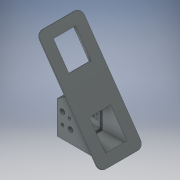
# Autodesk Inventor part: FingerScanTest
Saved by Autodesk Inventor 2017 (Build 210142000, 142)
## iProperties
Part Number: FingerScanTest
Material: Пластик АБС
Document SubType Name: Modeling
Designer: yulia_000
Density: 1.06 g/cm^3
Appearance: Цинк
Mass: 25.2515 g
Surface Area: 166.652 cm^2
Volume: 23.8222 cm^3
Author: yulia_000
Autodesk Inventor part; units mm, degrees
ref_plane "YZ Plane" through (0, 0, 0) normal (1, 0, 0) x (0, 1, 0)
sketch "Эскиз1" plane through (0, 0, 0) normal (0, 0, 1) x (1, 0, 0)
  line L0 (0, 25.2) -> (20.185268, 25.2)
  line L1 (20.185268, 25.2) -> (20.185268, 23.5) construction
  line L2 (20.185268, 23.5) -> (22.685268, 23.5) construction
  line L3 (22.685268, 23.5) -> (22.685268, 25.2) construction
  line L4 (31.435268, 25.2) -> (47.4, 2.4)
  line L5 (47.4, 2.4) -> (47.4, 0)
  line L6 (47.4, 0) -> (0, 0)
  line L7 (22.685268, 25.2) -> (31.435268, 25.2)
  line L8 (0, 25.2) -> (0, 0)
  line L9 (20.185268, 25.2) -> (22.685268, 25.2)
  point P0 (21.435268, 23.5)
  dimension "d2" = 2.4
  dimension "d8" = 1.7
  dimension "d10" = 47.4
  dimension "d13" = 25.2
  dimension "d34" = 35
  dimension "d37" = 2.5
  dimension "d38" = 10
  constraints: 21 end point, 6 perpendicular, 1 collinear, 1 horizontal, 1 midpoint, 1 parallel, 1 point on line, 1 vertical alignment
  measures "d2" distance of L4.end L5.end
  measures "d8" distance of L0.end L1.end
  measures "d10" distance of L5.end L6.end
  measures "d13" distance between parallel lines of L6 L0
  measures "d34" angle of L4 L5
  measures "d37" distance between parallel lines of L3 L1
  measures "d38" horizontal distance of L4.start point (21.435, 23.5)
extrude "Выдавливание1" add sketch "Эскиз1" along normal mid plane 21
shell "Оболочка1" thickness 3.8 outward yes removed faces 1 at (42.078423, 10, 3.5)
sketch "Эскиз7" plane through (-3.8, 29, 14.3) normal (0, 1, 0) x (1, 0, 0)
  line L0 (32.574479, 0) -> (0, 0)
  line L1 (0, 28.6) -> (32.574479, 28.6)
  line L2 (24.535268, 2) -> (27.435268, 2)
  line L3 (27.435268, 2) -> (27.435268, 26.6)
  line L4 (27.435268, 26.6) -> (24.535268, 26.6)
  line L5 (24.535268, 26.6) -> (24.535268, 2)
  line L6 (35.235268, 3.8) -> (35.235268, 24.8)
  point P0 (3.8, 14.3)
  dimension "d40" = 7.8
  dimension "d41" = 2
  dimension "d42" = 2
  dimension "d43" = 2.9
  constraints: 8 end point, 2 parallel, 1 horizontal, 1 perpendicular
  measures "d40" distance between parallel lines of L6 L3
  measures "d41" distance between parallel lines of L1 L4
  measures "d42" distance between parallel lines of L0 L2
  measures "d43" distance between parallel lines of L3 L5
extrude "Выдавливание7" cut sketch "Эскиз7" against normal blind 29
sketch "Эскиз8" plane through (0, 0, 14.3) normal (0, 0, 1) x (1, 0, 0)
  line L0 (51.2, -3.8) -> (51.2, -3.026962)
  line L1 (51.2, -3.8) -> (51.741287, -3.8)
  line L2 (51.2, -3.026962) -> (51.741287, -3.8)
  point P0 (0, 0)
  dimension "d46" = 35
  constraints: 4 end point, 1 horizontal
  measures "d46" angle of L0 L2
extrude "Выдавливание8" add sketch "Эскиз8" against normal blind 28.6
sketch "Эскиз10" plane through (0, 0, 14.3) normal (0, 0, 1) x (1, 0, 0)
  line L0 (-3.8, -3.8) -> (51.741287, -3.8)
  line L1 (52.667314, -6.691607) -> (50.64259, -3.8)
  line L2 (28.774479, 29) -> (-3.8, 29)
  line L3 (-10.124775, 84.553893) -> (-10.943927, 83.980316)
  line L4 (-10.943927, 83.980316) -> (27.553705, 29)
  line L5 (53.404551, -6.175388) -> (52.667314, -6.691607)
  line L6 (51.741287, -3.8) -> (28.774479, 29)
  line L7 (50.64259, -3.8) -> (51.741287, -3.8)
  line L8 (27.553705, 29) -> (28.774479, 29)
  line L9 (-3.8, 29) -> (28.774479, 29)
  line L10 (-10.124775, 84.553893) -> (28.774479, 29)
  line L11 (51.741287, -3.8) -> (53.404551, -6.175388)
  point P0 (0, 0)
  point P1 (23.635268, 29)
  dimension "d62" = 1
  dimension "d123" = 3.53
  dimension "d124" = 0.9
  dimension "d126" = 110.76
  constraints: 16 end point, 4 parallel, 2 collinear, 2 point on line, 1 perpendicular
  measures "d62" distance of L3.start L3.end
  measures "d123" distance of L1.start L1.end
  measures "d124" distance between parallel lines of L1 L6
  measures "d126" distance between parallel lines of L3 L5
extrude "Выдавливание9" add sketch "Эскиз10" against normal blind 28.6 contours L0 L11 L5 L1
extrude "Выдавливание10" add sketch "Эскиз10" against normal blind 28.6 contours L2 L4 L3 L10
sketch "Эскиз14" plane through (0, 0, 14.3) normal (0, 0, 1) x (1, 0, 0)
  line L0 (53.404551, -6.175388) -> (-10.124775, 84.553893)
  line L1 (-10.124775, 84.553893) -> (-10.943927, 83.980316)
  line L2 (27.553705, 29) -> (-10.943927, 83.980316)
  line L3 (53.404551, -6.175388) -> (52.667314, -6.691607)
  line L4 (-10.943927, 83.980316) -> (52.585399, -6.748964)
  line L5 (52.667314, -6.691607) -> (53.404551, -6.175388)
  line L6 (53.404551, -6.175388) -> (-10.124775, 84.553893)
  line L7 (-10.124775, 84.553893) -> (-10.943927, 83.980316)
  point P0 (0, 0)
  constraints: 8 end point, 1 collinear, 1 perpendicular
sketch "Эскиз14 outline for Выдавливание13" plane through (0, 0, 14.3) normal (0, 0, 1) x (1, 0, 0)
  line L0 (-10.943927, 83.980316) -> (52.667314, -6.691607)
  line L1 (-10.124775, 84.553893) -> (-10.943927, 83.980316)
  line L2 (53.404551, -6.175388) -> (-10.124775, 84.553893)
  line L3 (52.667314, -6.691607) -> (53.404551, -6.175388)
extrude "Выдавливание13" add sketch "Эскиз14 outline for Выдавливание13" along normal blind 8
sketch "Эскиз15" plane through (0, 0, -14.3) normal (0, 0, -1) x (-1, 0, 0)
  line L0 (10.943927, 83.980316) -> (10.124775, 84.553893)
  line L1 (10.124775, 84.553893) -> (-53.404551, -6.175388)
  line L2 (-53.404551, -6.175388) -> (-52.667314, -6.691607)
  line L3 (10.943927, 83.980316) -> (-52.667314, -6.691607)
  line L4 (-52.667314, -6.691607) -> (-53.404551, -6.175388)
  line L5 (-53.404551, -6.175388) -> (10.124775, 84.553893)
  line L6 (10.943927, 83.980316) -> (10.124775, 84.553893)
  point P0 (0, 0)
  constraints: 8 end point, 2 collinear, 1 perpendicular
extrude "Выдавливание14" add sketch "Эскиз15" along normal blind 8
fillet "Сопряжение2" radius 6 2 edges at (53.0359, -6.4335, 22.3) (53.0359, -6.4335, -22.3)
sketch "Эскиз16" plane through (0, 0, -10.5) normal (1, 0, 0) x (0, 0, -1)
  line L0 (-21, 0) -> (0, 0) projected
  line L1 (0, 0) -> (0, 25.2) projected
  line L2 (0, 25.2) -> (-21, 25.2) projected
  line L3 (-21, 25.2) -> (-21, 0) projected
  point P0 (-10.5, 0)
extrude "Выдавливание15" cut sketch "Эскиз16" against normal through all
sketch "Эскиз19" plane through (-3.8, -3.8, 14.3) normal (-1, 0, 0) x (0, 0, 1)
  line L0 (-24.8, 3.8) -> (-24.8, 29) projected
  line L1 (-24.8, 29) -> (-3.8, 29) projected
  line L2 (-3.8, 29) -> (-3.8, 3.8) projected
  line L3 (-3.8, 3.8) -> (-24.8, 3.8) projected
  line L4 (-3.55, 29.25) -> (-25.05, 29.25)
  line L5 (-25.05, 29.25) -> (-25.05, 3.55)
  line L6 (-25.05, 3.55) -> (-3.55, 3.55)
  line L7 (-3.55, 3.55) -> (-3.55, 29.25)
  point P0 (-14.3, 3.8)
  dimension "d106" = 0.25
  constraints: 8 end point, 3 other
  measures "d106" distance between parallel lines of L1 L4
extrude "Выдавливание17" cut sketch "Эскиз19" against normal up to surface (51.2 mm away)
sketch "Эскиз20" plane through (20.735268, 0, -12.3) normal (0, 1, 0) x (1, 0, 0)
  line L0 (0, -1.55) -> (2.9, -1.55) projected
  line L1 (2.9, 0) -> (2.9, -1.55) projected
  line L2 (0, 0) -> (2.9, 0) projected
  line L3 (0, -1.55) -> (0, 0) projected
  line L4 (2.9, -23.05) -> (0, -23.05) projected
  line L5 (0, -24.6) -> (0, -23.05) projected
  line L6 (2.9, -24.6) -> (0, -24.6) projected
  line L7 (2.9, -23.05) -> (2.9, -24.6) projected
  point P0 (-20.735268, -12.3)
extrude "Выдавливание18" cut sketch "Эскиз20" against normal up to surface (0.25 mm away)
sketch "Эскиз21" plane through (47.4, -0.25, -10.75) normal (-1, 0, 0) x (0, 0, 1)
  line L0 (0, 2.65) -> (21.5, 2.65) projected
  line L1 (0, 2.65) -> (0, 0) projected
  line L2 (0, 0) -> (21.5, 0) projected
  line L3 (21.5, 0) -> (21.5, 2.65) projected
  point P0 (10.75, 0.25)
extrude "Выдавливание19" cut sketch "Эскиз21" against normal blind 0.2
sketch "Эскиз22" plane through (-3.8, -3.8, 14.3) normal (-1, 0, 0) x (0, 0, 1)
  line L0 (-3.55, 29.25) -> (-3.55, 3.55) projected
  line L1 (-3.55, 3.55) -> (-25.05, 3.55) projected
  line L2 (-25.05, 3.55) -> (-25.05, 29.25) projected
  line L3 (-25.05, 29.25) -> (-3.55, 29.25) projected
  line L4 (0, 0) -> (-28.6, 0) projected
  line L5 (0, 32.8) -> (0, 0) projected
  line L6 (-28.6, 32.8) -> (0, 32.8) projected
  line L7 (-28.6, 0) -> (-28.6, 32.8) projected
  point P0 (-14.3, 3.8)
extrude "Выдавливание20" cut sketch "Эскиз22" against normal blind 6
sketch "Эскиз23" plane through (20.735268, -0.25, 12.3) normal (0, 1, 0) x (1, 0, 0)
  line L0 (-18.535268, 26.6) -> (-18.535268, -2)
  line L1 (6.818437, -2) -> (-18.535268, -2)
  line L2 (6.818437, -2) -> (6.818437, 26.6)
  line L3 (-18.535268, 26.6) -> (6.818437, 26.6)
  line L4 (2.9, 24.6) -> (2.9, 0)
  line L5 (2.9, 0) -> (0, 0)
  line L6 (0, 0) -> (0, 24.6)
  line L7 (0, 24.6) -> (2.9, 24.6)
  point P0 (-20.735268, 12.3)
extrude "Выдавливание21" cut sketch "Эскиз23" against normal through all contours L4 L5 L6 L7
sketch "Эскиз24" plane through (23.635268, 29, -12.3) normal (-1, 0, 0) x (0, 0, 1)
  line L0 (1.55, -3.55) -> (23.05, -3.55) projected
  line L1 (0, 0) -> (0, -32.8) projected
  line L2 (24.6, 0) -> (24.6, -32.8) projected
  line L3 (0, 0) -> (24.6, 0) projected
  line L4 (23.05, -3.55) -> (24.6, -3.55)
  line L5 (1.55, -3.55) -> (0, -3.55)
  point P0 (12.3, -29)
  constraints: 4 end point, 3 point on line, 1 perpendicular
extrude "Выдавливание22" add sketch "Эскиз24" along normal blind 3.8
fillet "Сопряжение4" radius 6 2 edges at (-10.5344, 84.2671, 22.3) (-10.5344, 84.2671, -22.3)
sketch "Эскиз25" plane through (52.667314, -6.691607, -16.3) normal (-0.819152, -0.5735764, 0) x (0, 0, 1)
  line L0 (30.6, 43.641427) -> (2, 43.641427)
  line L1 (2, 43.641427) -> (2, 104.13)
  line L2 (2, 104.13) -> (30.6, 104.13)
  line L3 (30.6, 104.13) -> (30.6, 43.641427)
  arc A0 (32.6, 0) -> (38.6, 6) centre (32.6, 6) ccw
  line L4 (0, 0) -> (32.6, 0)
  line L5 (5, 43.641427) -> (5, 101.13)
  line L6 (5, 101.13) -> (27.6, 101.13)
  line L7 (27.6, 101.13) -> (27.6, 43.641427)
  line L8 (2, 58.183715) -> (2, 43.641427)
  line L9 (2, 43.641427) -> (5, 43.641427)
  line L10 (30.6, 43.641427) -> (30.6, 58.183715)
  line L11 (27.6, 43.641427) -> (30.6, 43.641427)
  point P0 (16.3, 35.690174)
  dimension "d122" = 104.13
  dimension "d127" = 3
  dimension "d128" = 3
  dimension "d129" = 3
  constraints: 16 end point, 6 point on line, 4 perpendicular, 3 vertical, 1 horizontal
  measures "d122" distance between parallel lines of L2 L4
  measures "d127" distance between parallel lines of L1 L5
  measures "d128" distance between parallel lines of L3 L7
  measures "d129" distance between parallel lines of L2 L6
extrude "Выдавливание23" add sketch "Эскиз25" along normal blind 4 contours L0 L7 L6 L5 L1 L2 L3
sketch "Эскиз27" plane through (53.404551, -6.175388, 16.3) normal (0.819152, 0.5735764, 0) x (0, 0, -1)
  line L0 (5, 101.13) -> (27.6, 101.13)
  line L1 (5, 43.641427) -> (5, 101.13)
  line L2 (27.6, 101.13) -> (27.6, 43.641427)
  line L3 (3.5, 102.63) -> (3.5, 72.63)
  line L4 (3.5, 72.63) -> (29.1, 72.63)
  line L5 (29.1, 72.63) -> (29.1, 102.63)
  line L6 (3.5, 102.63) -> (29.1, 102.63)
  point P0 (16.3, 35.690174)
  dimension "d132" = 30
  dimension "d133" = 1.5
  dimension "d134" = 1.5
  dimension "d135" = 1.5
  constraints: 8 end point, 3 perpendicular, 1 parallel
  measures "d132" distance of L3.start L3.end
  measures "d133" distance between parallel lines of L2 L5
  measures "d134" distance between parallel lines of L3 L1
  measures "d135" distance between parallel lines of L6 L0
extrude "Выдавливание24" cut sketch "Эскиз27" against normal blind 1
sketch "Эскиз29" plane through (27.63562, 29.057358, -11.3) normal (-0.819152, -0.5735764, 0) x (0, 0, 1)
  line L0 (22.6, 28.988573) -> (0, 28.988573)
  line L1 (0, 28.988573) -> (0, 0)
  line L2 (22.6, 0) -> (0, 0)
  line L3 (22.6, 0) -> (22.6, 28.988573)
  point P0 (11.3, -7.951253)
extrude "Выдавливание25" add sketch "Эскиз29" along normal up to surface (4 mm away)
sketch "Эскиз30" plane through (11.745695, 53.319625, 12.8) normal (-0.5735764, 0.819152, 0) x (0.819152, 0.5735764, 0)
  line L0 (-4.9, 24.1) -> (-1, 24.1) projected
  line L1 (-4.9, 24.1) -> (-4.9, 1.5) projected
  line L2 (-1, 1.5) -> (-4.9, 1.5) projected
  line L3 (-1, 24.1) -> (-1, 1.5)
  point P0 (-40.20439, 12.8)
  constraints: 2 end point, 1 perpendicular
extrude "Выдавливание26" add sketch "Эскиз30" along normal blind 1
sketch "Эскиз31" plane through (20.735268, -0.25, -10.75) normal (0, 0, 1) x (1, 0, 0)
  line L0 (0, 0) -> (0, 25.7)
  line L1 (-18.535268, 25.7) -> (0, 25.7)
  line L2 (-16.535268, 25.7) -> (0, 2.08519) construction
  line L3 (-16.535268, 25.7) -> (5.761904, 25.7) construction
  line L4 (-15.81421, 23.7) -> (-10.11421, 23.7)
  line L5 (-10.11421, 23.7) -> (-10.11421, 17.5)
  line L6 (-10.11421, 17.5) -> (-15.81421, 17.5)
  line L7 (-15.81421, 17.5) -> (-15.81421, 23.7)
  line L8 (-15.81421, 23.7) -> (-10.11421, 17.5) construction
  line L9 (-10.11421, 23.7) -> (-15.81421, 17.5) construction
  line L10 (-7.7, 5.911708) -> (-2, 5.911708)
  line L11 (-2, 5.911708) -> (-2, 12.111708)
  line L12 (-2, 12.111708) -> (-7.7, 12.111708)
  line L13 (-7.7, 12.111708) -> (-7.7, 5.911708)
  line L14 (-7.7, 5.911708) -> (-2, 12.111708) construction
  line L15 (-2, 5.911708) -> (-7.7, 12.111708) construction
  point P0 (-20.735268, 0.25)
  point P1 (-12.96421, 20.6)
  point P2 (-4.85, 9.011708)
  dimension "d144" = 55
  dimension "d145" = 2
  dimension "d147" = 5.7
  dimension "d148" = 6.2
  dimension "d149" = 2
  dimension "d150" = 5.7
  dimension "d151" = 6.2
  dimension "d152" = 2
  constraints: 28 end point, 4 midpoint, 4 parallel, 4 point on line, 3 horizontal, 2 perpendicular
  measures "d144" angle of L2 L3
  measures "d145" distance of L2.start L1.start
  measures "d147" distance of L5.end L6.end
  measures "d148" distance of L4.end L5.end
  measures "d149" distance between parallel lines of L1 L4
  measures "d150" distance of L12.end L11.end
  measures "d151" distance of L11.end L10.end
  measures "d152" distance between parallel lines of L0 L11
extrude "Выдавливание27" cut sketch "Эскиз31" against normal blind 2 contours L4 L5 L6 L7
extrude "Выдавливание28" cut sketch "Эскиз31" against normal blind 2 contours L13 L12 L11 L10
hole "Отверстие2" at (7.771058, 20.35, -10.75) direction (0, 0, -1) diameter 3 end through all
hole "Отверстие3" at (15.885268, 8.761708, -10.75) direction (0, 0, -1) diameter 3 end through all
sketch "Эскиз32" plane through (0, 0, -14.3) normal (0, 0, -1) x (-1, 0, 0)
  circle A0 centre (-15.885268, 8.761708) radius 1.5
  circle A1 centre (-7.771058, 20.35) radius 1.5
  line L0 (7.141115, 78.549338) -> (10.943927, 83.980316)
  line L1 (10.943927, 83.980316) -> (-50.638696, -3.8)
  line L2 (-50.638696, -3.8) -> (-2.2, -3.8)
  line L3 (-2.2, -3.8) -> (-2.2, 29)
  line L4 (-2.2, 29) -> (-22.792684, 29)
  line L5 (10.335808, 76.31239) -> (-22.792684, 29)
  line L6 (7.141115, 78.549338) -> (10.335808, 76.31239)
  line L7 (-0.710638, 30.413974) -> (-58.142216, -51.449411)
  line L8 (-49.221418, -1.779802) -> (7.498031, 79.068511)
  line L9 (218.905608, 88.550589) -> (-81.094392, 88.550589)
  line L10 (-58.142216, -51.449411) -> (171.857784, -51.449411)
  point P0 (0, 0)
  dimension "d171" = 100
  dimension "d172" = 140
  dimension "d173" = 230
  constraints: 5 end point, 1 horizontal, 1 parallel, 1 point on line
  measures "d171" distance of L7.end L7.start
  measures "d172" distance between parallel lines of L10 L9
  measures "d173" distance of L7.end L10.end
sketch "Эскиз33" plane through (0, 0, -14.3) normal (0, 0, -1) x (-1, 0, 0)
  circle A0 centre (-15.885268, 8.761708) radius 1.5
  circle A1 centre (-7.771058, 20.35) radius 1.5
  line L0 (7.141115, 78.549338) -> (10.943927, 83.980316)
  line L1 (10.943927, 83.980316) -> (-50.638696, -3.8)
  line L2 (-50.638696, -3.8) -> (-2.2, -3.8)
  line L3 (-2.2, -3.8) -> (-2.2, 29)
  line L4 (-2.2, 29) -> (-22.792684, 29)
  line L5 (10.335808, 76.31239) -> (-22.792684, 29)
  line L6 (7.141115, 78.549338) -> (10.335808, 76.31239)
  line L7 (173.443902, -47.988783) -> (-72.354853, -47.988783)
  line L8 (22.8, -47.988783) -> (22.8, 27.011217)
  point P0 (0, 0)
  dimension "d174" = 25
  dimension "d175" = 75
  constraints: 2 end point, 1 point on line, 1 vertical
  measures "d174" distance between parallel lines of L3 L8
  measures "d175" distance of L8.start L8.end
ref_plane "РабПлоскость4" through (-22.8, 27.011217, -14.3) normal (1, 0, 0) x (0, 0, 1)
ref_plane "РабПлоскость3" through (-32.8, 27.011217, -14.3) normal (1, 0, 0) x (0, 0, 1)
sketch "Эскиз35" plane through (-22.8, 27.011217, -14.3) normal (1, 0, 0) x (0, 0, 1)
  line L0 (-20, 0) -> (-20, 75)
  line L1 (48.6, 0) -> (48.6, 75)
  line L2 (-20, 0) -> (48.6, 0)
  line L3 (0, 30.811217) -> (0, -1.988783)
  point P0 (14.3, 27.011217)
  point P1 (14.3, 0)
  constraints: 2 end point, 1 midpoint, 1 perpendicular
ref_plane "РабПлоскость5" through (5.357497, 29.884708, -17.3) normal (0, 0, -1) x (0.8186339, 0.5743158, 0)
sketch "Эскиз36" plane through (5.357497, 29.884708, -17.3) normal (0, 0, -1) x (0.8186339, 0.5743158, 0)
  line L0 (0, 51.39476) -> (-55, 51.39476)
  line L1 (0, 1.080713) -> (0, 95.126155)
  line L2 (-179.265703, -49.938847) -> (6.5, 80.385807)
  point P0 (-21.549088, 21.387739)
  dimension "d176" = 20
  dimension "d177" = 55
  constraints: 2 end point, 1 perpendicular, 1 point on line
  measures "d176" distance from line of L0.start L2
  measures "d177" distance of L0.start L0.end
sketch "Эскиз37" plane through (0, 0, 14.3) normal (0, 0, 1) x (1, 0, 0)
  line L0 (22.792684, 29) -> (2.2, 29)
  line L1 (22.792684, 29) -> (-10.335808, 76.31239)
  line L2 (16.017898, 38.675397) -> (2.2, 29)
  point P0 (0, 0)
  constraints: 2 end point, 1 perpendicular, 1 point on line
extrude "Выдавливание29" add sketch "Эскиз37" against normal up to surface (28.6 mm away)
sketch "Эскиз38" plane through (52.585399, -6.748964, 16.3) normal (0.819152, 0.5735764, 0) x (0, 0, -1)
  line L0 (5, 73.63) -> (5, 101.13) projected
  line L1 (5, 101.13) -> (27.6, 101.13) projected
  line L2 (27.6, 101.13) -> (27.6, 73.63) projected
  line L3 (5, 73.63) -> (27.6, 73.63) projected
  line L4 (29.1, 72.63) -> (3.5, 72.63) projected
  line L5 (29.1, 102.63) -> (29.1, 72.63) projected
  line L6 (3.5, 102.63) -> (29.1, 102.63) projected
  line L7 (3.5, 72.63) -> (3.5, 102.63) projected
  point P0 (16.3, 35.690174)
extrude "Выдавливание30" cut sketch "Эскиз38" against normal blind 10
extrude "Выдавливание31" add sketch "Эскиз38" along normal up to surface (1 mm away)
sketch "Эскиз39" plane through (20.735268, -0.25, 10.75) normal (0, 0, -1) x (-1, 0, 0)
  line L0 (18.535268, 25.7) -> (0, 25.7) construction
  line L1 (18.535268, 0) -> (0, 0) construction
  line L2 (10.11421, 23.7) -> (10.11421, 17.5) construction
  line L3 (10.11421, 17.5) -> (15.81421, 17.5) construction
  circle A0 centre (12.96421, 20.6) radius 1.5 construction
  line L4 (15.81421, 17.5) -> (15.81421, 23.7) construction
  line L5 (15.81421, 23.7) -> (10.11421, 23.7) construction
  line L6 (7.7, 12.111708) -> (2, 12.111708) construction
  line L7 (7.7, 5.911708) -> (7.7, 12.111708) construction
  circle A1 centre (4.85, 9.011708) radius 1.5 construction
  line L8 (2, 5.911708) -> (7.7, 5.911708) construction
  line L9 (2, 12.111708) -> (2, 5.911708) construction
  line L10 (8.907105, 25.7) -> (8.907105, 0)
  circle A2 centre (12.96421, 20.6) radius 2.5
  circle A3 centre (4.85, 9.011708) radius 2.5
  line L11 (8.907105, 21.2) -> (8.907105, 15)
  line L12 (8.907105, 15) -> (3.207105, 15)
  circle A4 centre (6.057105, 18.1) radius 1.5
  line L13 (3.207105, 15) -> (3.207105, 21.2)
  line L14 (3.207105, 21.2) -> (8.907105, 21.2)
  line L15 (10.11421, 12.111708) -> (15.81421, 12.111708)
  line L16 (10.11421, 5.911708) -> (10.11421, 12.111708)
  circle A5 centre (12.96421, 9.011708) radius 1.5
  line L17 (15.81421, 5.911708) -> (10.11421, 5.911708)
  line L18 (15.81421, 12.111708) -> (15.81421, 5.911708)
  point P0 (20.735268, 0.25)
  point P1 (8.907105, 18.1)
  point P2 (6.057105, 15)
  dimension "d185" = 5
  dimension "d186" = 5
  dimension "d203" = 6.2
  dimension "d204" = 5.7
  dimension "d216" = 15
  dimension "d218" = 2.41421
  constraints: 18 end point, 5 symmetric about line, 4 centre point, 3 parallel, 3 point on line, 2 coincident, 2 midpoint, 1 equal radius, 1 horizontal alignment, 1 vertical, 1 vertical alignment, 1 other
  measures "d185" diameter of A2
  measures "d186" diameter of A3
  measures "d203" distance of L13.start L13.end
  measures "d204" distance of L13.end L14.end
  measures "d216" distance between parallel lines of L1 L12
  measures "d218" diameter of L2 L10
extrude "Выдавливание32" cut sketch "Эскиз39" against normal through all contours A2 | A3 | A4 | A5
extrude "Выдавливание33" cut sketch "Эскиз39" against normal blind 2 contours L10 L12 L13 L14 | L15 L18 L17 L16
